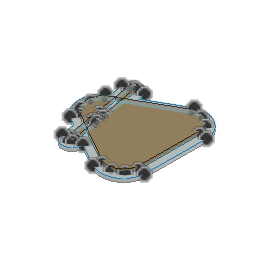
logo terre vorace (Autodesk Fusion 360 design; units mm, degrees)
Autodesk Fusion 360 part; units mm, degrees
sketch "Esquisse1" plane through (0, 0, 0) normal (0, 1, 0) x (1, 0, 0)
sketch "Esquisse2" plane through (0, 0, 0) normal (0, 1, 0) x (1, 0, 0)
  line L0 (-7.1984, 5.7929) -> (5.54, 13.0097)
  line L1 (12.224, 8.699) -> (12.1271, -9.222)
  line L2 (5.2978, -12.903) -> (-5.0189, -7.0424)
  line L3 (-5.0189, -7.0424) -> (-4.4376, -10.7234)
  line L4 (-5.9876, -11.014) -> (-6.8594, -5.9768)
  line L5 (-6.8594, -5.9768) -> (-10.3467, -3.8457)
  line L6 (-10.6857, 3.807) -> (-8.6999, 5.0179)
  line L7 (-8.6999, 5.0179) -> (-9.6202, 10.0067)
  line L8 (-7.1984, 5.7929) -> (-8.0703, 10.2973)
  line L9 (-8.6999, 5.0179) -> (-7.1984, 5.7929)
  line L10 (-6.8594, -5.9768) -> (-5.0189, -7.0424)
  line L11 (-5.0189, -7.0424) -> (-5.4827, -4.0424)
  line L12 (-6.8594, -5.9768) -> (-7.1185, -4.1951)
  line L13 (-8.6999, 5.0179) -> (-7.7946, -0.5527)
  line L14 (-7.1984, 5.7929) -> (-6.2024, -0.2692)
  spline S0 degree 5 poles (-10.6857, 3.807) (-10.7699, 3.7194) (-10.9329, 3.5405) (-11.1609, 3.262) (-11.4318, 2.8699) (-11.7139, 2.345) (-11.9372, 1.7861) (-12.0992, 1.1967) (-12.1982, 0.5832) (-12.2336, -0.0425) (-12.2055, -0.6652) (-12.1151, -1.2686) (-11.9635, -1.8369) (-11.7524, -2.3571) (-11.4841, -2.8215) (-11.1611, -3.227) (-10.8608, -3.5037) (-10.6126, -3.6849) (-10.437, -3.794) (-10.3467, -3.8457) knots 0 0 0 0 0 0 0.066667 0.133333 0.2 0.266667 0.333333 0.4 0.466667 0.533333 0.6 0.666667 0.733333 0.8 0.866667 0.933333 1 1 1 1 1 1
  spline S1 degree 5 poles (-5.9876, -11.014) (-5.98, -11.0815) (-5.962, -11.211) (-5.9262, -11.389) (-5.8609, -11.5936) (-5.7497, -11.7934) (-5.6098, -11.9361) (-5.4437, -12.0212) (-5.2571, -12.05) (-5.0595, -12.0267) (-4.8639, -11.9579) (-4.6838, -11.8508) (-4.5321, -11.7128) (-4.4193, -11.5504) (-4.3509, -11.3682) (-4.3292, -11.1692) (-4.3494, -10.998) (-4.3855, -10.8632) (-4.4187, -10.7705) (-4.4376, -10.7234) knots 0 0 0 0 0 0 0.066667 0.133333 0.2 0.266667 0.333333 0.4 0.466667 0.533333 0.6 0.666667 0.733333 0.8 0.866667 0.933333 1 1 1 1 1 1
  spline S2 degree 5 poles (-9.6202, 10.0067) (-9.6184, 10.0519) (-9.6131, 10.1401) (-9.5997, 10.2658) (-9.5709, 10.4199) (-9.5164, 10.5894) (-9.4434, 10.7347) (-9.3521, 10.854) (-9.2441, 10.9456) (-9.1223, 11.0075) (-8.9906, 11.0379) (-8.8533, 11.0351) (-8.7144, 10.9979) (-8.577, 10.9258) (-8.443, 10.8194) (-8.3135, 10.6798) (-8.2137, 10.5424) (-8.1411, 10.4253) (-8.0937, 10.341) (-8.0703, 10.2973) knots 0 0 0 0 0 0 0.066667 0.133333 0.2 0.266667 0.333333 0.4 0.466667 0.533333 0.6 0.666667 0.733333 0.8 0.866667 0.933333 1 1 1 1 1 1
  spline S3 degree 5 poles (-7.7946, -0.5527) (-7.7612, -0.6069) (-7.6946, -0.7105) (-7.595, -0.8519) (-7.463, -1.012) (-7.2995, -1.1638) (-7.138, -1.2662) (-6.9798, -1.3193) (-6.8266, -1.3244) (-6.6815, -1.2859) (-6.5481, -1.2112) (-6.4304, -1.1085) (-6.3323, -0.9864) (-6.2568, -0.8522) (-6.2053, -0.7111) (-6.1784, -0.5661) (-6.1761, -0.4483) (-6.1851, -0.359) (-6.1959, -0.2992) (-6.2024, -0.2692) knots 0 0 0 0 0 0 0.066667 0.133333 0.2 0.266667 0.333333 0.4 0.466667 0.533333 0.6 0.666667 0.733333 0.8 0.866667 0.933333 1 1 1 1 1 1
  spline S4 degree 5 poles (-7.1185, -4.1951) (-7.1273, -4.1462) (-7.1416, -4.0505) (-7.1525, -3.9136) (-7.1458, -3.7446) (-7.1017, -3.5566) (-7.0219, -3.3935) (-6.9082, -3.2574) (-6.7647, -3.1513) (-6.5991, -3.0788) (-6.421, -3.0438) (-6.2407, -3.0501) (-6.0678, -3.1006) (-5.9095, -3.1972) (-5.77, -3.3397) (-5.6512, -3.5272) (-5.5732, -3.712) (-5.5243, -3.8698) (-5.4958, -3.9835) (-5.4827, -4.0424) knots 0 0 0 0 0 0 0.066667 0.133333 0.2 0.266667 0.333333 0.4 0.466667 0.533333 0.6 0.666667 0.733333 0.8 0.866667 0.933333 1 1 1 1 1 1
  spline S5 degree 5 poles (5.54, 13.0097) (5.6415, 13.057) (5.8467, 13.1442) (6.1609, 13.2531) (6.5927, 13.3541) (7.1534, 13.4049) (7.733, 13.3783) (8.3266, 13.273) (8.925, 13.0897) (9.5138, 12.8319) (10.0763, 12.5047) (10.5954, 12.1138) (11.0555, 11.665) (11.4452, 11.1636) (11.7593, 10.6142) (11.9964, 10.0205) (12.1249, 9.512) (12.1875, 9.1125) (12.2143, 8.8382) (12.224, 8.699) knots 0 0 0 0 0 0 0.066667 0.133333 0.2 0.266667 0.333333 0.4 0.466667 0.533333 0.6 0.666667 0.733333 0.8 0.866667 0.933333 1 1 1 1 1 1
  spline S6 degree 5 poles (12.1271, -9.222) (12.1122, -9.3477) (12.0761, -9.5956) (12.0029, -9.957) (11.8667, -10.4177) (11.6309, -10.9569) (11.3289, -11.4568) (10.961, -11.9136) (10.5308, -12.3221) (10.0458, -12.6759) (9.5162, -12.9679) (8.9528, -13.1911) (8.3662, -13.3397) (7.7651, -13.4101) (7.155, -13.4017) (6.5396, -13.3162) (6.0444, -13.1875) (5.6716, -13.058) (5.4225, -12.9571) (5.2978, -12.903) knots 0 0 0 0 0 0 0.066667 0.133333 0.2 0.266667 0.333333 0.4 0.466667 0.533333 0.6 0.666667 0.733333 0.8 0.866667 0.933333 1 1 1 1 1 1
  line L15 (-5.7636, 8.9045) -> (-6.1644, 10.9757)
  spline S7 degree 3 poles (-11.6273, 9.8625) (-11.6244, 9.9366) (-11.6215, 10.0106) (-11.6187, 10.0847) (-11.5981, 10.6109) (-11.5086, 11.1908) (-11.1328, 11.7914) (-10.8094, 12.3082) (-10.2251, 12.7973) (-9.519, 12.9643) (-8.8485, 13.1228) (-8.1086, 12.9653) (-7.5907, 12.6581) (-6.9707, 12.2904) (-6.6308, 11.8133) (-6.3692, 11.3538) (-6.3483, 11.3172) (-6.328, 11.2804) (-6.3082, 11.2434) (-6.2603, 11.1542) (-6.2124, 11.065) (-6.1644, 10.9757) knots -0.065512 -0.065512 -0.065512 -0.065512 0 0 0 0.267845 0.267845 0.267845 0.498306 0.498306 0.498306 0.717136 0.717136 0.717136 0.979101 0.979101 0.979101 1 1 1 1.081691 1.081691 1.081691 1.081691
  line L16 (-10.9165, 6.0088) -> (-11.6273, 9.8625)
  line L17 (-11.9486, 5.3795) -> (-10.9165, 6.0088)
  spline S8 degree 3 poles (-11.9486, 5.3795) (-12.0085, 5.3171) (-12.0684, 5.2547) (-12.1284, 5.1923) (-13.1498, 4.1285) (-13.8529, 2.7498) (-14.1047, 1.2701) (-14.3725, -0.3036) (-14.196, -1.9549) (-13.4657, -3.359) (-12.9883, -4.2766) (-12.2497, -5.0545) (-11.3675, -5.5657) knots -0.028469 -0.028469 -0.028469 -0.028469 0 0 0 0.361544 0.361544 0.361544 0.746051 0.746051 0.746051 0.997343 0.997343 0.997343 0.997343
  line L18 (-8.6755, -7.2108) -> (-11.3675, -5.5657)
  line L19 (-7.9672, -11.3033) -> (-8.6755, -7.2108)
  spline S9 degree 3 poles (-7.9672, -11.3033) (-7.9089, -11.7699) (-7.8016, -12.2574) (-7.48, -12.777) (-7.2137, -13.2071) (-6.7471, -13.6451) (-6.1942, -13.8602) (-5.5957, -14.0931) (-4.9994, -14.068) (-4.525, -13.9431) (-3.8951, -13.7771) (-3.3791, -13.4541) (-2.9579, -12.9299) (-2.5662, -12.4424) (-2.3301, -11.744) (-2.3414, -11.1207) (-2.343, -11.0299) (-2.3489, -10.9406) (-2.3583, -10.854) knots 0.008172 0.008172 0.008172 0.008172 0.179714 0.179714 0.179714 0.321692 0.321692 0.321692 0.475411 0.475411 0.475411 0.679585 0.679585 0.679585 0.869444 0.869444 0.869444 0.897086 0.897086 0.897086 0.897086
  line L20 (4.4033, -14.6951) -> (-2.3583, -10.854)
  spline S10 degree 3 poles (14.1265, -9.3452) (14.1221, -9.3824) (14.1177, -9.4196) (14.1133, -9.4569) (13.9484, -10.8507) (13.3861, -12.1991) (12.4284, -13.2435) (11.2723, -14.5046) (9.608, -15.2956) (7.8758, -15.3872) (6.7194, -15.4484) (5.5728, -15.2024) (4.5018, -14.7378) (4.469, -14.7236) (4.4361, -14.7093) (4.4033, -14.6951) knots -0.011842 -0.011842 -0.011842 -0.011842 0 0 0 0.331858 0.331858 0.331858 0.732526 0.732526 0.732526 1 1 1 1.010536 1.010536 1.010536 1.010536
  line L21 (14.2244, 8.7631) -> (14.1265, -9.3452)
  spline S11 degree 3 poles (4.6236, 14.7892) (4.6477, 14.8004) (4.6718, 14.8116) (4.696, 14.8229) (5.9988, 15.4293) (7.5313, 15.5394) (8.9662, 15.1545) (10.3979, 14.7705) (11.7739, 13.9432) (12.7601, 12.7117) (13.6356, 11.6185) (14.1212, 10.2454) (14.2192, 8.8378) (14.2209, 8.8129) (14.2226, 8.788) (14.2244, 8.7631) knots -0.009504 -0.009504 -0.009504 -0.009504 0 0 0 0.346802 0.346802 0.346802 0.692835 0.692835 0.692835 1 1 1 1.007161 1.007161 1.007161 1.007161
  line L22 (-5.7636, 8.9045) -> (4.6236, 14.7892)
  point P0 (-12.1008, 1.1081)
  point P1 (-11.8883, -1.9946)
  point P2 (-5.4039, -12.0173)
  point P3 (-4.534, -11.6977)
  point P4 (-9.3358, 10.8596)
  point P5 (-8.7483, 11.0014)
  point P6 (-6.9047, -1.3161)
  point P7 (-6.3172, -0.9514)
  point P8 (-6.9028, -3.2668)
  point P9 (-6.1132, -3.0951)
  point P10 (8.1681, 13.2894)
  point P11 (10.9712, 11.7249)
  point P12 (10.9712, -11.8733)
  point P13 (8.4289, -13.3075)
  dimension "d3" = -2
extrude "Extrusion1" add sketch "Esquisse2" along normal blind 1 contours L7 L8 L9 S2 | L0 L1 L2 L5 L6 L11 L12 L13 L14 S0 S3 S4 S5 S6 | L3 L4 L10 S1 makes body 1 at (6.2735, 0, 1.4601)
extrude "Extrusion2" add sketch "Esquisse2" against normal blind 1 separate body contours L7 L8 L9 S2 | L9 L13 L14 S3 | L0 L1 L2 L5 L6 L11 L12 L13 L14 S0 S3 S4 S5 S6 | L3 L4 L10 S1 | L10 L11 L12 S4 | L15 S7 L16 L17 S8 L18 L19 S9 L20 S10 L21 S11 L22 makes body 2
combine "Combiner1" operation add target body 2 tool bodies 1
